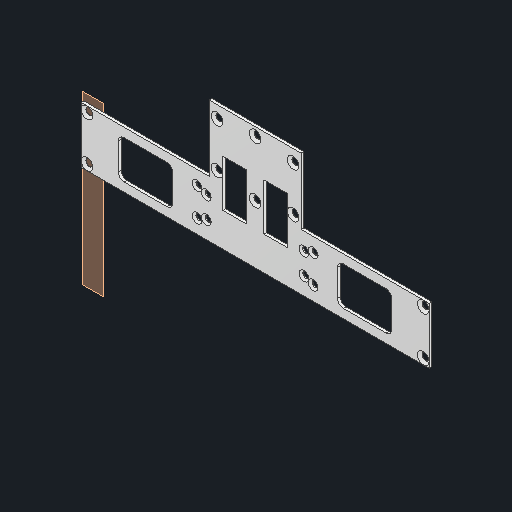
# Autodesk Inventor part: ceil
Saved by Autodesk Inventor 2023 (Build 270158000, 158)
## iProperties
Created: 2024-04-25
Part Number: ceil
Material: ABS Plastic
Document SubType Name: Modeling
Designer: szymo
Density: 1.06 g/cm^3
Appearance: Smooth - White
Mass: 7.10721 g
Surface Area: 110.803 cm^2
Volume: 6.70491 cm^3
Author: szymo
Autodesk Inventor part; units mm, degrees
ref_plane "YZ Plane" through (0, 0, 0) normal (1, 0, 0) x (0, 1, 0)
ref_plane "XZ Plane" through (0, 0, 0) normal (0, 1, 0) x (-1, 0, 0)
ref_plane "XY Plane" through (0, 0, 0) normal (0, 0, 1) x (1, 0, 0)
ref_plane "Work Plane1" through (0, 0, 0) normal (0, 0, 1) x (1, 0, 0)
ref_plane "Work Plane2" through (0, 0, 0) normal (0, 0, 1) x (1, 0, 0)
sketch "Sketch3" plane through (0, 0, 0) normal (0, 0, 1) x (1, 0, 0)
  circle A0 centre (3, -25.75) radius 2.3 projected
  circle A1 centre (3, -3) radius 2.3 projected
  circle A2 centre (3, -74.8889) radius 2.3 projected
  line L0 (0, 0) -> (6, 0) projected
  line L1 (0, -77.8889) -> (0, 0) projected
  line L2 (0, -77.8889) -> (6, -77.8889) projected
  line L3 (6, -71.8889) -> (6, -77.8889) projected
  line L4 (6, -71.8889) -> (1.6, -71.8889) projected
  line L5 (1.6, -71.8889) -> (1.6, -56.7889) projected
  line L6 (1.6, -56.7889) -> (9.6, -56.7889) projected
  line L7 (9.6, -44.7889) -> (9.6, -56.7889) projected
  line L8 (3, -44.7889) -> (9.6, -44.7889) projected
  line L9 (3, -28.75) -> (3, -44.7889) projected
  line L10 (3, -28.75) -> (6, -28.75) projected
  line L11 (6, -28.75) -> (6, -22.75) projected
  line L12 (6, -22.75) -> (3, -22.75) projected
  line L13 (3, -6) -> (3, -22.75) projected
  line L14 (3, -6) -> (6, -6) projected
  line L15 (6, -6) -> (6, 0) projected
  circle A3 centre (5.6, -52.7889) radius 2.6 projected
  circle A4 centre (175, -3) radius 2.3 projected
  circle A5 centre (175, -25.75) radius 2.3 projected
  line L16 (175, -28.75) -> (175, -41.8889) projected
  line L17 (168.4, -41.8889) -> (175, -41.8889) projected
  line L18 (168.4, -53.8889) -> (168.4, -41.8889) projected
  line L19 (175, -53.8889) -> (168.4, -53.8889) projected
  line L20 (175, -53.8889) -> (175, -71.8889) projected
  line L21 (172, -71.8889) -> (172, -77.8889) projected
  line L22 (178, -77.8889) -> (172, -77.8889) projected
  line L23 (178, -77.8889) -> (178, 0) projected
  line L24 (178, 0) -> (172, 0) projected
  line L25 (172, 0) -> (172, -6) projected
  line L26 (172, -6) -> (175, -6) projected
  line L27 (175, -6) -> (175, -22.75) projected
  line L28 (175, -22.75) -> (172, -22.75) projected
  line L29 (172, -22.75) -> (172, -28.75) projected
  line L30 (172, -28.75) -> (175, -28.75) projected
  circle A6 centre (175, -74.8889) radius 2.3 projected
  circle A7 centre (172.4, -49.8889) radius 2.6 projected
  circle A8 centre (89, 0.9661) radius 2.3 projected
  circle A9 centre (89, 29.5) radius 2.3 projected
  circle A10 centre (89, 15.55) radius 3.3 projected
  circle A11 centre (89, -14.375) radius 3.3 projected
  circle A12 centre (89, 41.2) radius 3.3 projected
  line L31 (93.5, -27.75) -> (84.5, -27.75) projected
  line L32 (93.5, 55) -> (93.5, -27.75) projected
  line L33 (84.5, 55) -> (93.5, 55) projected
  line L34 (84.5, -27.75) -> (84.5, 55) projected
  line L35 (105.5, -27.75) -> (111.5, -27.75) projected
  line L36 (111.5, -24.9105) -> (111.5, -27.75) projected
  arc A13 (105.5, -24.9105) -> (111.5, -24.9105) centre (108.5, -23.95) ccw projected
  line L37 (105.5, -27.75) -> (105.5, -24.9105) projected
  arc A14 (111.5, -22.9895) -> (105.5, -22.9895) centre (108.5, -23.95) ccw projected
  line L38 (111.5, -5.5855) -> (111.5, -22.9895) projected
  arc A15 (105.5, -5.5855) -> (111.5, -5.5855) centre (108.5, -4.625) ccw projected
  line L39 (105.5, -22.9895) -> (105.5, -5.5855) projected
  circle A16 centre (108.4846, 4.5875) radius 2.3 projected
  arc A17 (105.5, 12.8395) -> (111.5, 12.8395) centre (108.5, 13.8) ccw projected
  line L40 (105.5, -3.6645) -> (105.5, 12.8395) projected
  arc A18 (111.5, -3.6645) -> (105.5, -3.6645) centre (108.5, -4.625) ccw projected
  line L41 (111.5, 12.8395) -> (111.5, -3.6645) projected
  circle A19 centre (108.4462, 27.5) radius 2.3 projected
  arc A20 (111.5, 14.7605) -> (105.5, 14.7605) centre (108.5, 13.8) ccw projected
  line L42 (111.5, 40.6331) -> (111.5, 14.7605) projected
  arc A21 (105.5, 40.1338) -> (111.5, 40.6331) centre (108.4231, 41.3077) ccw projected
  line L43 (105.5, 14.7605) -> (105.5, 40.1338) projected
  arc A22 (111.5, 41.9823) -> (105.5, 42.4816) centre (108.4231, 41.3077) ccw projected
  line L44 (111.5, 55) -> (111.5, 41.9823) projected
  line L45 (105.5, 55) -> (111.5, 55) projected
  line L46 (105.5, 42.4816) -> (105.5, 55) projected
  line L47 (111.5, 41.9823) -> (111.5, 55) projected
  line L48 (111.5, 41.9823) -> (112.5, 41.9823) projected
  line L49 (112.5, 41.9823) -> (112.5, 55) projected
  line L50 (111.5, 55) -> (112.5, 55) projected
  line L51 (111.5, 14.7605) -> (111.5, 40.6331) projected
  line L52 (111.5, 14.7605) -> (112.5, 14.7605) projected
  line L53 (112.5, 14.7605) -> (112.5, 40.6331) projected
  line L54 (111.5, 40.6331) -> (112.5, 40.6331) projected
  line L55 (111.5, 0) -> (111.5, 12.8395) projected
  line L56 (112.5, 0) -> (112.5, 12.8395) projected
  line L57 (111.5, 12.8395) -> (112.5, 12.8395) projected
  line L58 (66.5, 14.7605) -> (66.5, 40.6331) projected
  line L59 (66.5, 40.6331) -> (65.5, 40.6331) projected
  line L60 (65.5, 14.7605) -> (65.5, 40.6331) projected
  line L61 (66.5, 14.7605) -> (65.5, 14.7605) projected
  line L62 (66.5, 41.9823) -> (66.5, 55) projected
  line L63 (66.5, 55) -> (65.5, 55) projected
  line L64 (65.5, 41.9823) -> (65.5, 55) projected
  line L65 (66.5, 41.9823) -> (65.5, 41.9823) projected
  line L66 (66.5, 0) -> (66.5, 12.8395) projected
  line L67 (66.5, 12.8395) -> (65.5, 12.8395) projected
  line L68 (65.5, 0) -> (65.5, 12.8395) projected
  arc A23 (66.5, -5.5855) -> (72.5, -5.5855) centre (69.5, -4.625) ccw projected
  line L69 (66.5, -22.9895) -> (66.5, -5.5855) projected
  arc A24 (72.5, -22.9895) -> (66.5, -22.9895) centre (69.5, -23.95) ccw projected
  line L70 (72.5, -5.5855) -> (72.5, -22.9895) projected
  line L71 (66.5, -27.75) -> (72.5, -27.75) projected
  line L72 (72.5, -24.9105) -> (72.5, -27.75) projected
  arc A25 (66.5, -24.9105) -> (72.5, -24.9105) centre (69.5, -23.95) ccw projected
  line L73 (66.5, -27.75) -> (66.5, -24.9105) projected
  circle A26 centre (69.5, 4.5875) radius 2.3 projected
  arc A27 (72.5, -3.6645) -> (66.5, -3.6645) centre (69.5, -4.625) ccw projected
  line L74 (72.5, 12.8395) -> (72.5, -3.6645) projected
  arc A28 (66.5, 12.8395) -> (72.5, 12.8395) centre (69.5, 13.8) ccw projected
  line L75 (66.5, -3.6645) -> (66.5, 12.8395) projected
  circle A29 centre (69.5, 27.5) radius 2.3 projected
  arc A30 (66.5, 40.6331) -> (72.5, 40.1338) centre (69.5769, 41.3077) ccw projected
  line L76 (66.5, 14.7605) -> (66.5, 40.6331) projected
  arc A31 (72.5, 14.7605) -> (66.5, 14.7605) centre (69.5, 13.8) ccw projected
  line L77 (72.5, 40.1338) -> (72.5, 14.7605) projected
  arc A32 (72.5, 42.4816) -> (66.5, 41.9823) centre (69.5769, 41.3077) ccw projected
  line L78 (72.5, 55) -> (72.5, 42.4816) projected
  line L79 (66.5, 55) -> (72.5, 55) projected
  line L80 (66.5, 41.9823) -> (66.5, 55) projected
  circle A33 centre (59.3, -21.5445) radius 1.75 projected
  circle A34 centre (59.3, -7.2055) radius 1.75 projected
  line L81 (56.8, -28.75) -> (56.8, 0) projected
  line L82 (61.8, -28.75) -> (56.8, -28.75) projected
  line L83 (61.8, 0) -> (61.8, -28.75) projected
  line L84 (61.8, 0) -> (56.8, 0) projected
  circle A35 centre (64.05, -19.8657) radius 1.75 projected
  circle A36 centre (64.05, -8.8843) radius 1.75 projected
  line L85 (61.8, 0) -> (61.8, -28.75) projected
  line L86 (61.8, -28.75) -> (66.3, -28.75) projected
  line L87 (66.3, 0) -> (66.3, -28.75) projected
  line L88 (61.8, 0) -> (66.3, 0) projected
  circle A37 centre (113.95, -19.8657) radius 1.75 projected
  circle A38 centre (113.95, -8.8843) radius 1.75 projected
  line L89 (116.2, 0) -> (116.2, -28.75) projected
  line L90 (116.2, 0) -> (111.7, 0) projected
  line L91 (111.7, 0) -> (111.7, -28.75) projected
  line L92 (116.2, -28.75) -> (111.7, -28.75) projected
  circle A39 centre (118.7, -21.5445) radius 1.75 projected
  circle A40 centre (118.7, -7.2055) radius 1.75 projected
  line L93 (121.2, -28.75) -> (121.2, 0) projected
  line L94 (116.2, 0) -> (121.2, 0) projected
  line L95 (116.2, 0) -> (116.2, -28.75) projected
  line L96 (116.2, -28.75) -> (121.2, -28.75) projected
  line L97 (0, 0) -> (178, 0)
  line L98 (178, 0) -> (178, -28.75)
  line L99 (178, -28.75) -> (0, -28.75)
  line L100 (0, -28.75) -> (0, 0)
  line L101 (112.5, 0) -> (65.5, 0)
  line L102 (65.5, 0) -> (65.5, 55)
  line L103 (65.5, 55) -> (112.5, 55)
  line L104 (112.5, 55) -> (112.5, 0)
  line L105 (104.5, 11.4325) -> (104.5, -10.5675) projected
  line L106 (94.5, -10.5675) -> (94.5, 11.4325) projected
  line L107 (104.5, 11.4325) -> (73.5, 11.4325)
  line L108 (73.5, 11.4325) -> (73.5, -10.5675)
  line L109 (73.5, -10.5675) -> (104.5, -10.5675)
  line L110 (104.5, -10.5675) -> (104.5, 11.4325)
  line L111 (72.5, 12.4325) -> (105.5, 12.4325)
  line L112 (105.5, 12.4325) -> (105.5, -11.5675)
  line L113 (105.5, -11.5675) -> (72.5, -11.5675)
  line L114 (72.5, -11.5675) -> (72.5, 12.4325)
  line L115 (175, -71.8889) -> (172, -71.8889) projected
  arc A41 (22.05, -4.5875) -> (19.05, -7.5875) centre (22.05, -7.5875) ccw projected
  line L116 (22.05, -4.5875) -> (43.875, -4.5875) projected
  line L117 (19.05, -21.225) -> (19.05, -7.5875) projected
  arc A42 (19.05, -21.225) -> (22.05, -24.225) centre (22.05, -21.225) ccw projected
  line L118 (43.875, -24.225) -> (22.05, -24.225) projected
  arc A43 (43.875, -24.225) -> (46.875, -21.225) centre (43.875, -21.225) ccw projected
  line L119 (46.875, -7.5875) -> (46.875, -21.225) projected
  arc A44 (46.875, -7.5875) -> (43.875, -4.5875) centre (43.875, -7.5875) ccw projected
  line L120 (134.125, -4.525) -> (155.95, -4.525) projected
  arc A45 (158.95, -7.525) -> (155.95, -4.525) centre (155.95, -7.525) ccw projected
  line L121 (158.95, -7.525) -> (158.95, -21.1625) projected
  arc A46 (155.95, -24.1625) -> (158.95, -21.1625) centre (155.95, -21.1625) ccw projected
  line L122 (155.95, -24.1625) -> (134.125, -24.1625) projected
  arc A47 (131.125, -21.1625) -> (134.125, -24.1625) centre (134.125, -21.1625) ccw projected
  line L123 (131.125, -21.1625) -> (131.125, -7.525) projected
  arc A48 (134.125, -4.525) -> (131.125, -7.525) centre (134.125, -7.525) ccw projected
  line L124 (65.5, 33.8) -> (112.5, 33.8)
  line L125 (66.5, 0) -> (65.5, 0) projected
  line L126 (111.5, 0) -> (112.5, 0) projected
  point P0 (112.5, 0)
  point P1 (65.5, 0)
  point P2 (0, -28.75)
  point P3 (172, 0)
  point P4 (93.5, 12.4325)
  point P5 (105.5, -5.5855)
  point P6 (93.5, -11.5675)
  point P7 (84.5, -11.5675)
  point P8 (72.5, -5.5855)
  point P9 (84.5, 12.4325)
  point P10 (111.5, 33.8)
  dimension "d29" = 1
  dimension "d30" = 1
  dimension "d31" = 1
  dimension "d38" = 4.6
  dimension "d39" = 4.3
  constraints: 34 end point, 8 parallel, 7 point on line, 6 perpendicular, 3 horizontal, 3 other
  measures "d29" distance between parallel lines of L105 L40
  measures "d30" distance between parallel lines of L74 L108
  measures "d31" distance between parallel lines of L107 L111
  measures "d38" diameter of A9
  measures "d39" distance from line of L124 A9.centre
extrude "Extrusion2" add sketch "Sketch3" along normal blind 1.4 contours A0 | A1 | L0 L15 L14 L13 L12 L11 L10 L99 L1 | L97 L81 L99 L11 L12 L13 L14 L15 | L84 L83 L82 L81 | L88 L87 L86 L83 | L68 L67 L66 L97 L88 | L87 L97 L75 A27 L114 A23 L69 A24 L70 L113 L34 L31 L32 L39 A14 L38 A15 L112 A18 L41 L91 L99 | L102 L61 A31 L77 L124 L34 L111 L74 A28 L67 | L91 L90 L89 L92 | A28 L74 L97 L66 | L60 L124 L58 L61 | L97 L74 A27 L75 | L97 L41 L57 L56 L90 | L89 L94 L93 L96 | L58 L124 L77 A31 | L97 L40 A17 L41 | L41 A18 L40 L97 | L93 L97 L25 L26 L27 L28 L29 L99 | L57 A17 L40 L111 L32 L124 L43 A20 L52 L104 | L29 L28 L27 L26 L25 L24 L23 L99 L30 | L111 A10 L32 L107 L34 | L34 L124 L32 L111 A10 | L70 A24 L69 A23 | L97 A8 L32 L109 L34 | L34 L107 L32 L97 A8 | L52 L42 L124 L53 | L111 A10 | A10 L111 | L109 L32 L113 A11 L34 | L97 A8 | A8 L97 | A20 L43 L124 L42 | A15 L38 A14 L39 | L113 A11 L32 L31 L34 | L113 A11 | A11 L113 | A4 | A5 | A9 | L37 A13 L36 L35 | A16 | A19 | L73 A25 L72 L71 | A26 | A29 | A33 | A34 | A35 | A36 | A37 | A38 | A39 | A40
sketch "Sketch4" plane through (0, 0, 1.4) normal (0, 0, 1) x (1, 0, 0)
  circle A0 centre (69.5, 27.5) radius 2.3 projected
  circle A1 centre (69.5, 4.5875) radius 2.3 projected
  circle A2 centre (89, 0.9661) radius 2 projected
  circle A3 centre (89, 29.5) radius 2.3 projected
  circle A4 centre (108.4462, 27.5) radius 2.3 projected
  circle A5 centre (108.4846, 4.5875) radius 2.3 projected
  circle A6 centre (64.05, -8.8843) radius 1.75 projected
  circle A7 centre (59.3, -7.2055) radius 1.75 projected
  circle A8 centre (59.3, -21.5445) radius 1.75 projected
  circle A9 centre (64.05, -19.8657) radius 1.75 projected
  circle A10 centre (118.7, -21.5445) radius 1.75 projected
  circle A11 centre (113.95, -19.8657) radius 1.75 projected
  circle A12 centre (113.95, -8.8843) radius 1.75 projected
  circle A13 centre (118.7, -7.2055) radius 1.75 projected
  circle A14 centre (3, -25.75) radius 2.3 projected
  circle A15 centre (3, -3) radius 2.3 projected
  circle A16 centre (175, -25.75) radius 2.3 projected
  circle A17 centre (175, -3) radius 2.3 projected
  point P0 (0, 0)
  constraints: 18 coincident
hole "Hole2" at (3, -3, 1.4) at (3, -25.75, 1.4) at (175, -3, 1.4) at (175, -25.75, 1.4) at (108.4846, 4.5875, 1.4) at (89, 0.9661, 1.4) at (69.5, 4.5875, 1.4) at (69.5, 27.5, 1.4) at (89, 29.5, 1.4) at (108.4462, 27.5, 1.4) direction (0, 0, -1) diameter 3.6 end through all countersink diameter 6 countersink angle 90 clearance for "Countersunk Flat Head Screw ISO 2009/7046" size "M3" standard "ISO"
sketch "Sketch5" plane through (0, 0, 1.4) normal (0, 0, 1) x (1, 0, 0)
  circle A0 centre (64.05, -19.8657) radius 1.75 projected
  circle A1 centre (59.3, -21.5445) radius 1.75 projected
  circle A2 centre (59.3, -7.2055) radius 1.75 projected
  circle A3 centre (64.05, -8.8843) radius 1.75 projected
  circle A4 centre (113.95, -8.8843) radius 1.75 projected
  circle A5 centre (118.7, -7.2055) radius 1.75 projected
  circle A6 centre (118.7, -21.5445) radius 1.75 projected
  circle A7 centre (113.95, -19.8657) radius 1.75 projected
  point P0 (0, 0)
  constraints: 8 coincident
hole "Hole3" at (59.3, -7.2055, 1.4) at (64.05, -8.8843, 1.4) at (64.05, -19.8657, 1.4) at (59.3, -21.5445, 1.4) at (113.95, -8.8843, 1.4) at (118.7, -7.2055, 1.4) at (118.7, -21.5445, 1.4) at (113.95, -19.8657, 1.4) direction (0, 0, -1) diameter 3.1 end through all countersink diameter 5 countersink angle 90 clearance for "Countersunk Flat Head Screw ISO 2009/7046" size "M2.5" standard "ISO"
equation "\"d30\" = d29"
body "Solid2"
